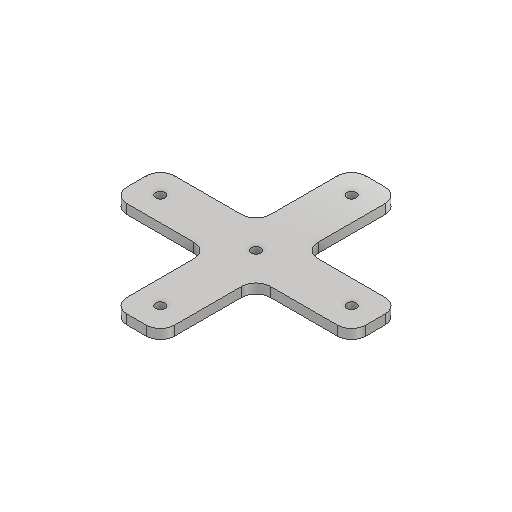
# Autodesk Inventor part: LC_ALU_4mm_Heatbed_Frame_X_Bracket
Saved by Autodesk Inventor 2026.1 (Build 301233000, 233)
## iProperties
Created: 2016-06-30
Part Number: LC_ALU_4mm_Heatbed_Frame_X_Bracket
Material: Ogólny
Document SubType Name: Modeling
Designer: Andrzej
Density: 1 g/cm^3
Appearance: Aluminium - polerowane
Author: Andrzej
Autodesk Inventor part; units mm, degrees
ref_plane "YZ Plane" through (0, 0, 0) normal (1, 0, 0) x (0, 1, 0)
ref_plane "XZ Plane" through (0, 0, 0) normal (0, 1, 0) x (-1, 0, 0)
ref_plane "XY Plane" through (0, 0, 0) normal (0, 0, 1) x (1, 0, 0)
sketch "Szkic1" plane through (0, 0, 0) normal (0, 0, 1) x (1, 0, 0)
  line L0 (-47.736, 26.7667) -> (-47.736, 6.7667)
  line L1 (-47.736, 26.7667) -> (52.264, 26.7667)
  line L2 (52.264, 26.7667) -> (52.264, 6.7667)
  circle A0 centre (-37.736, 16.7667) radius 2
  circle A1 centre (2.264, 16.7667) radius 2
  circle A2 centre (42.264, 16.7667) radius 2
  line L3 (-7.736, 26.7667) -> (-7.736, 66.7667)
  line L4 (-7.736, 66.7667) -> (12.264, 66.7667)
  line L5 (12.264, 66.7667) -> (12.264, 26.7667)
  circle A3 centre (2.264, 56.7667) radius 2
  line L6 (-47.736, 6.7667) -> (52.264, 6.7667)
  line L7 (-7.736, 6.7667) -> (-7.736, -33.2333)
  line L8 (-7.736, -33.2333) -> (12.264, -33.2333)
  line L9 (12.264, -33.2333) -> (12.264, 6.7667)
  circle A4 centre (2.264, -23.2333) radius 2
  point P0 (0, 0)
  dimension "d0" = 20
  dimension "d1" = 100
  dimension "d4" = 4
  dimension "d5" = 4
  dimension "d6" = 4
  dimension "d7" = 10
  dimension "d8" = 10
  dimension "d9" = 10
  dimension "d10" = 10
  dimension "d11" = 10
  dimension "d12" = 50
  dimension "d13" = 40
  dimension "d14" = 20
  dimension "d15" = 40
  dimension "d16" = 10
  dimension "d17" = 10
  dimension "d18" = 4
  dimension "d20" = 40
  dimension "d21" = 20
  dimension "d22" = 10
  dimension "d23" = 10
  dimension "d24" = 4
  constraints: 20 end point, 6 perpendicular, 5 centre point, 4 point on line, 2 coincident, 2 horizontal, 2 vertical
  measures "d0" distance of L1.start L0.end
  measures "d1" distance of L1.start L1.end
  measures "d4" diameter of A0
  measures "d5" diameter of A1
  measures "d6" diameter of A2
  measures "d7" distance from line of L0 A0.centre
  measures "d8" distance from line of L1 A0.centre
  measures "d9" distance from line of L1 A1.centre
  measures "d10" distance from line of L1 A2.centre
  measures "d11" distance from line of L2 A2.centre
  measures "d12" distance from line of L0 A1.centre
  measures "d13" distance of L3.start L3.end
  measures "d14" distance of L3.end L4.end
  measures "d15" distance between parallel lines of L0 L3
  measures "d16" distance from line of L3 point (2.264, 56.767)
  measures "d17" distance from line of point (2.264, 56.767) L4
  measures "d18" diameter of A3
  measures "d20" distance of L7.start L7.end
  measures "d21" distance of L7.end L8.end
  measures "d22" distance from line of L8 point (2.264, -23.233)
  measures "d23" distance from line of L7 point (2.264, -23.233)
  measures "d24" diameter of A4
extrude "Wyciągnięcie proste1" add sketch "Szkic1" along normal blind 4
fillet "Zaokrąglenie1" radius 6 12 edges at (12.264, 26.7667, 2) (-7.736, 6.7667, 2) (-7.736, 26.7667, 2) (-47.736, 26.7667, 2) (-47.736, 6.7667, 2) (12.264, 66.7667, 2) (-7.736, 66.7667, 2) (52.264, 26.7667, 2) (52.264, 6.7667, 2) (12.264, 6.7667, 2) (12.264, -33.2333, 2) (-7.736, -33.2333, 2)
equation "\"d12\" = 0.5 * d1"
equation "\"d22\" = d17"
equation "\"d23\" = d16"
